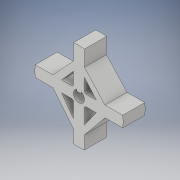
# Autodesk Inventor part: Spokes2
Saved by Autodesk Inventor 2017 (Build 210142000, 142)
## iProperties
Created: 2016-12-01
Part Number: Spokes2
Material: Generic
Document SubType Name: Modeling
Designer: JJ
Density: 1 g/cm^3
Appearance: Default
Author: JJ
Autodesk Inventor part; units mm, degrees
ref_plane "YZ Plane" through (0, 0, 0) normal (1, 0, 0) x (0, 1, 0)
ref_plane "XZ Plane" through (0, 0, 0) normal (0, 1, 0) x (-1, 0, 0)
ref_plane "XY Plane" through (0, 0, 0) normal (0, 0, 1) x (1, 0, 0)
sketch "Sketch1" plane through (0, 0, 0) normal (0, 0, 1) x (1, 0, 0)
  circle A0 centre (0, 0) radius 6.35
  circle A1 centre (0, 0) radius 10
  arc A2 (6.35, 50.4016) -> (-6.35, 50.4016) centre (0, 0) ccw
  arc A3 (50.4016, -6.35) -> (50.4016, 6.35) centre (0, 0) ccw
  arc A4 (-6.35, -50.4016) -> (6.35, -50.4016) centre (0, 0) ccw
  arc A5 (-50.4016, 6.35) -> (-50.4016, -6.35) centre (0, 0) ccw
  line L0 (6.35, -35.2008) -> (30, -6.35)
  line L1 (30, 6.35) -> (6.35, 32.112)
  line L2 (-6.35, 32.112) -> (-30, 6.35)
  line L3 (-30, -6.35) -> (-6.35, -35.2008)
  line L4 (-6.35, -25.2008) -> (-20, -6.35)
  line L5 (-20, 6.35) -> (-6.35, 22.112)
  line L6 (6.35, 22.112) -> (20, 6.35)
  line L7 (20, -6.35) -> (6.35, -25.2008)
  line L8 (20, -6.35) -> (7.7251, -6.35)
  line L9 (7.7251, 6.35) -> (20, 6.35)
  line L10 (6.35, 22.112) -> (6.35, 7.7251)
  line L11 (-6.35, 22.112) -> (-6.35, 7.7251)
  line L12 (-7.7251, 6.35) -> (-20, 6.35)
  line L13 (-7.7251, -6.35) -> (-20, -6.35)
  line L14 (-6.35, -25.2008) -> (-6.35, -7.7251)
  line L15 (6.35, -7.7251) -> (6.35, -25.2008)
  line L16 (7.7251, -6.35) -> (20, -6.35)
  line L17 (20, 6.35) -> (7.7251, 6.35)
  line L18 (-6.35, 7.7251) -> (-6.35, 22.112)
  line L19 (6.35, 7.7251) -> (6.35, 22.112)
  line L20 (-30, 6.35) -> (-50.4016, 6.35)
  line L21 (-50.4016, -6.35) -> (-30, -6.35)
  line L22 (-6.35, -35.2008) -> (-6.35, -50.4016)
  line L23 (6.35, -50.4016) -> (6.35, -35.2008)
  line L24 (30, -6.35) -> (50.4016, -6.35)
  line L25 (50.4016, 6.35) -> (30, 6.35)
  line L26 (6.35, 32.112) -> (6.35, 50.4016)
  line L27 (-6.35, 32.112) -> (-6.35, 50.4016)
  line L28 (-0.0474, 3.8498) -> (2.5, 3.8498)
  line L29 (-0.0474, 3.8498) -> (-2.5, 3.8498)
  line L30 (2.5, 3.8498) -> (2.5, 5.8372)
  line L31 (-2.5, 3.8498) -> (-2.5, 5.8372)
  dimension "d0" = 12.7
  dimension "d6" = 40
  dimension "d7" = 10
  dimension "d8" = 10
  dimension "d9" = 10
  dimension "d10" = 10
  constraints: 64 end point, 10 point on circle, 7 parallel, 6 perpendicular, 5 centre point, 2 coincident, 1 horizontal, 1 point on line, 1 vertical, 10 other
  measures "d0" diameter of A0
  measures "d6" distance of L6.end L5.start
  measures "d7" distance of L4.end L3.start
  measures "d8" distance of L5.end L2.start
  measures "d9" distance of L0.end L7.start
  measures "d10" distance of L3.end L4.start
extrude "Extrusion1" add sketch "Sketch1" along normal blind 25.4 contours L30 L28 L29 L31 A0 | A1 | L26 L1 L25 A3 L24 L0 L23 A4 L22 L3 L21 A5 L20 L2 L27 A2 picked at (1.2429, 4.64)
body "Solid1"
